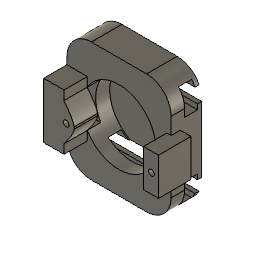
Gear_Box (Autodesk Fusion 360 design; units mm, degrees)
part number: 2026-08-12-20-34-04-092
Autodesk Fusion 360 part; units mm, degrees
sketch "Sketch3" plane through (0, 0, 0) normal (0, 1, 0) x (1, 0, 0)
  line L0 (9, -19.5) -> (-9, -19.5)
  line L1 (-17, -11.5) -> (-17, 11.5)
  line L2 (-9, 19.5) -> (9, 19.5)
  line L3 (17, 11.5) -> (17, -11.5)
  line L4 (17, -19.5) -> (-17, 19.5) construction
  line L5 (-17, -19.5) -> (17, 19.5) construction
  arc A0 (9, -19.5) -> (17, -11.5) centre (9, -11.5) ccw
  arc A1 (-17, -11.5) -> (-9, -19.5) centre (-9, -11.5) ccw
  arc A2 (-9, 19.5) -> (-17, 11.5) centre (-9, 11.5) ccw
  arc A3 (17, 11.5) -> (9, 19.5) centre (9, 11.5) ccw
  dimension "d25" = 39
  dimension "d26" = 34
  dimension "d41" = 8
  dimension "d42" = 8
  dimension "d43" = 8
  dimension "d44" = 8
  constraint horizontal L0
  constraint perpendicular L0 L1
  constraint parallel L0 L2
  constraint parallel L1 L3
  constraint coincident L4 origin
  constraint coincident L5 origin
  constraint coincident L4.start L3
  constraint coincident L4.start L0
  constraint tangent L3 A0
  constraint tangent L0 A0
  constraint coincident L5.start L0
  constraint coincident L5.start L1
  constraint tangent L0 A1
  constraint tangent L1 A1
  constraint equal A0 A1
  constraint coincident L4.end L1
  constraint coincident L4.end L2
  constraint tangent L1 A2
  constraint tangent L2 A2
  constraint equal A0 A2
  constraint coincident L5.end L2
  constraint coincident L5.end L3
  constraint tangent L2 A3
  constraint tangent L3 A3
  measures "d25" distance of L4.start L5.end
  measures "d26" distance of L4.end L5.end
  measures "d41" radius of A0
  measures "d42" radius of A3
  measures "d43" radius of A2
  measures "d44" radius of A1
extrude "Extrude3" add sketch "Sketch3" along normal blind 10
sketch "Sketch4" plane through (-17, 0, 0) normal (-1, 0, 0) x (0, -1, 0)
  line L0 (0, -11.5) -> (0, 11.5)
  line L1 (-10, 11.5) -> (-10, -11.5)
  line L2 (-8.6, -16.7) -> (-4.4, -16.7)
  line L3 (-4.4, -16.7) -> (-4.4, -9.05)
  line L4 (-4.4, -9.05) -> (-8.6, -9.05)
  line L5 (-10, -10.75) -> (-10, -15)
  line L6 (-10, 0) -> (0, 0) construction
  line L7 (-8.6, -16.7) -> (-8.6, -15)
  line L8 (-8.6, -15) -> (-10, -15)
  line L9 (-4.4, -12.875) -> (-10, -12.875) construction
  line L10 (-8.6, -9.05) -> (-8.6, -10.75)
  line L11 (-8.6, -10.75) -> (-10, -10.75)
  line L12 (0, 11.5) -> (-10, 11.5)
  line L13 (-10, -11.5) -> (0, -11.5)
  point P0 (0, -19.5)
  dimension "d50" = 4.2
  constraint horizontal L2
  constraint vertical L3
  constraint horizontal L4
  constraint vertical L5
  constraint midpoint L1 L6.start
  constraint coincident L6.end origin
  constraint vertical L7
  constraint horizontal L8
  constraint midpoint L3 L9.start
  constraint symmetric L2.start L9 L4.end
  constraint symmetric L7.end L9 L10.end
  constraint symmetric L5.end L9 L5.start
  constraint coincident L5 L9.end
  measures "d50" distance of L2.end L2.start
extrude "Extrude4" cut sketch "Sketch4" against normal blind 34 contours L1 L3 L4 L5 L10 L11 L13 | L2 L3 L5 L7 L8 L13
mirror "Mirror1" about plane through (0, 0, 0) normal (0, 0, 1) of "Extrude4"
sketch "Sketch5" plane through (0, 0, 0) normal (0, -1, 0) x (1, 0, 0)
  line L0 (-9, -19.5) -> (9, -19.5)
  line L1 (17, -11.5) -> (17, 11.5)
  line L2 (9, 19.5) -> (-9, 19.5)
  line L3 (-17, 11.5) -> (-17, -11.5)
  circle A0 centre (0, 0) radius 12
  arc A1 (17, 11.5) -> (9, 19.5) centre (9, 11.5) ccw
  arc A2 (-9, 19.5) -> (-17, 11.5) centre (-9, 11.5) ccw
  arc A3 (-17, -11.5) -> (-9, -19.5) centre (-9, -11.5) ccw
  arc A4 (9, -19.5) -> (17, -11.5) centre (9, -11.5) ccw
  line L4 (17, -6.1) -> (-17, -6.1)
  line L5 (-17, -6.1) -> (-17, 6.1)
  line L6 (-17, 6.1) -> (17, 6.1)
  line L7 (-7, 6.1) -> (-7, -6.1) construction
  line L8 (-7, 6.1) -> (-7, -6.1)
  circle A5 centre (-9.6, 0) radius 0.95
  line L9 (4.3, 6.1) -> (4.3, -6.1) construction
  circle A6 centre (18.2, 0) radius 0.95
  line L10 (17, -6.1) -> (20.5, -6.1)
  line L11 (20.5, -6.1) -> (20.5, 6.1)
  line L12 (20.5, 6.1) -> (17, 6.1)
  line L13 (-11.2949, -4.0529) -> (-7, -2.5118) construction
  line L14 (11.2949, 4.0529) -> (17, 6.1) construction
  line L15 (15.6, 6.1) -> (15.6, -6.1)
  point P0 (-7, 0)
  dimension "d38" = 24
  dimension "d51" = 12.2
  dimension "d52" = 7
  dimension "d57" = 1.9
  dimension "d58" = 2.6
  dimension "d61" = 11.3
  dimension "d62" = 30.1
  dimension "d63" = 4.9
  constraint coincident A0.centre origin
  constraint horizontal L4
  constraint perpendicular L4 L5
  constraint parallel L4 L6
  constraint coincident A0.centre L14
  constraint coincident L1 L4.start
  constraint midpoint L7 P0
  constraint coincident L4 L7.end
  constraint perpendicular L4 L7
  constraint coincident L6 L9.start
  constraint coincident L4 L9.end
  constraint perpendicular L4 L9
  constraint symmetric A5 L9 A6
  constraint horizontal L10
  constraint vertical L11
  constraint horizontal L12
  constraint coincident A0 L13.start
  constraint coincident L7 L13.end
  constraint collinear L13 L14
  constraint coincident A0 L14.start
  constraint coincident L6 L15.start
  constraint coincident L4 L15.end
  constraint perpendicular L4 L15
  measures "d38" diameter of A0
  measures "d51" distance of L4.start L6.end
  measures "d52" distance of A0.centre L7
  measures "d57" diameter of A5
  measures "d58" distance of P0 A5.centre
  measures "d61" distance of L8 L9
  measures "d62" distance of A5.centre L11
  measures "d63" distance of L11 L15
extrude "Extrude6" cut sketch "Sketch5" against normal blind 4.4 contours L3 A0 L4 L5 L6
extrude "Extrude7" add sketch "Sketch5" against normal blind 2 contours A0 L4 L6 L8 | A5 picked at (-9.102, 3.8855)
extrude "Extrude8" cut sketch "Sketch5" against normal blind 6 contours A5
extrude "Extrude9" add sketch "Sketch5" along normal blind 6 contours L3 A0 L4 L5 L6 | L1 L4 L6 L15 | L1 L10 L11 L12 | A0 L4 L6 L8 picked at (-9.102, 3.8855)
extrude "Extrude5" cut sketch "Sketch5" against normal blind 9 contours A0 L4 | A0 L4 L6 L8 | A0 L6 | A0 L4 L6 L8 | A5
move_face "OffsetFaces1" offset 3 1 faces at (18.5903, 0, 4.3824)
sketch "Sketch6" plane through (0, -6, 0) normal (0, -1, 0) x (1, 0, 0)
  circle A0 centre (-9.6, 0) radius 0.95
  line L0 (-7, 6.1) -> (-17, 6.1)
  line L1 (-17, 6.1) -> (-17, -6.1)
  line L2 (-17, -6.1) -> (-7, -6.1)
  line L3 (-7, -6.1) -> (-7, 6.1)
  line L4 (-10.3185, 6.1) -> (-10.3185, -6.1)
  spline S0 degree 2 poles (-10.3185, 6.1) (-5.8098, 0) (-10.3185, -6.1) knots 0 0 0 1.390569 1.390569 1.390569 weights 1 2.846154 1
  constraint coincident L0 L4.start
  constraint coincident L2 L4.end
  constraint perpendicular L2 L4
extrude "Extrude10" cut sketch "Sketch6" against normal blind 6 contours L0 L3 S0 | L2 L3 S0
extrude "Extrude11" add 1 faces at (-12.5508, -4, -6.1) along direction (0, 0, -1) blind 3
extrude "Extrude12" add 1 faces at (-12.5508, -4, 6.1) along direction (0, 0, 1) blind 3
extrude "Extrude13" add 2 faces at (-14.85, -6, 0) (18.0763, -6, 4.3824) along direction (0, -1, 0) blind 1.6
